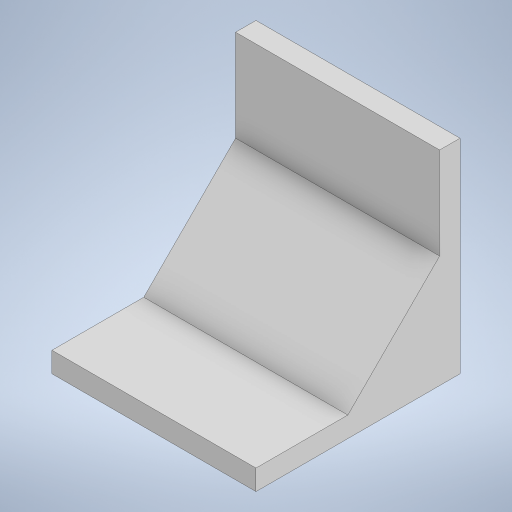
# Autodesk Inventor part: 肋
Saved by Autodesk Inventor 2024.2 (Build 282272000, 272)
## iProperties
Created: 2024-05-02
Part Number: 肋
Material: 一般
Document SubType Name: Modeling
Designer: User
Density: 1 g/cm^3
Appearance: 預設
Author: User
Autodesk Inventor part; units mm, degrees
ref_plane "YZ Plane" through (0, 0, 0) normal (1, 0, 0) x (0, 1, 0)
ref_plane "XZ Plane" through (0, 0, 0) normal (0, 1, 0) x (-1, 0, 0)
ref_plane "XY Plane" through (0, 0, 0) normal (0, 0, 1) x (1, 0, 0)
sketch "草圖1" plane through (0, 0, 0) normal (1, 0, 0) x (0, 1, 0)
  line L0 (0, 0) -> (1, 0)
  line L1 (1, 0) -> (1, 10)
  line L2 (1, 10) -> (0, 10)
  line L3 (0, 10) -> (0, 0)
  line L4 (0, 0) -> (10, 0)
  line L5 (10, 0) -> (10, 1)
  line L6 (10, 1) -> (0, 1)
  line L7 (0, 1) -> (0, 0)
  point P0 (1, 1)
  dimension "d0" = 1
  dimension "d1" = 10
  dimension "d2" = 10
  dimension "d3" = 1
  constraints: 16 end point, 4 parallel, 2 horizontal, 2 perpendicular
  measures "d0" distance of L2.end L1.end
  measures "d1" distance of L1.end L0.end
  measures "d2" distance of L6.end L5.end
  measures "d3" distance of L5.end L4.end
extrude "擠出1" add sketch "草圖1" along normal blind 5 and the other way blind 5
sketch "草圖3" plane through (0, 0, 0) normal (1, 0, 0) x (0, 1, 0)
  line L0 (1, 1) -> (1, 10) projected
  line L1 (1, 5.5) -> (5.5, 1)
  line L2 (10, 1) -> (1, 1) projected
  point P0 (0, 0)
  dimension "d9" = 45
  constraints: 2 end point, 2 midpoint
  measures "d9" angle of L2 L1
extrude "肋1" add sketch "草圖3" along normal mid plane 10 rib yes fills toward (3.2146, 3.2146) open curves L1
